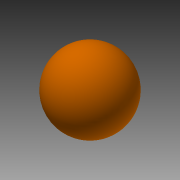
# Autodesk Inventor part: Bola Pingpong
Saved by Autodesk Inventor 2015 (Build 190159000, 159)
## iProperties
Created: 2015-02-08
Part Number: Bola Pingpong
Material: Generic
Document SubType Name: Modeling
Designer: Rafi Kurnia Putra
Density: 1 g/cm^3
Appearance: Default
Mass: 33.5103 g
Surface Area: 50.2655 cm^2
Volume: 33.5103 cm^3
Author: Rafi Kurnia Putra
Autodesk Inventor part; units mm, degrees
ref_plane "YZ Plane" through (0, 0, 0) normal (1, 0, 0) x (0, 1, 0)
ref_plane "XZ Plane" through (0, 0, 0) normal (0, 1, 0) x (-1, 0, 0)
ref_plane "XY Plane" through (0, 0, 0) normal (0, 0, 1) x (1, 0, 0)
sketch "Sketch1" plane through (0, 0, 0) normal (0, 1, 0) x (-1, 0, 0)
  line L0 (20, 0) -> (-20, 0)
  line L1 (20, 0) -> (60, 0) construction
  arc A0 (20, 0) -> (-20, 0) centre (0, 0) ccw
  dimension "d0" = 40
  dimension "d1" = 180
  dimension "d2" = 40
  constraints: 4 end point, 2 horizontal, 2 point on circle, 1 centre point, 1 coincident, 1 collinear
  measures "d0" distance of L0.start L0.end
  measures "d1" angle of L0 L1
  measures "d2" diameter of A0
revolve "Revolution1" add sketch "Sketch1" angle 360 about axis through (-20, 0, 0) along (1, 0, 0)
body "Solid1"
